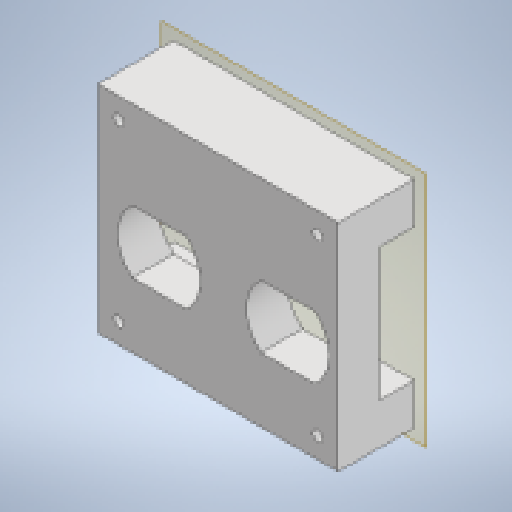
# Autodesk Inventor part: house_V5
Saved by Autodesk Inventor 2023 (Build 270158000, 158)
## iProperties
Created: 2023-03-13
Part Number: house_V5
Material: Generic
Document SubType Name: Modeling
Designer: shrey
Density: 1 g/cm^3
Appearance: Default
Author: shrey
Autodesk Inventor part; units mm, degrees
ref_plane "YZ Plane" through (0, 0, 0) normal (1, 0, 0) x (0, 1, 0)
ref_plane "XZ Plane" through (0, 0, 0) normal (0, 1, 0) x (-1, 0, 0)
ref_plane "XY Plane" through (0, 0, 0) normal (0, 0, 1) x (1, 0, 0)
ref_plane "Work Plane1" through (-29.0856, -229.9846, 23.749) normal (0, 0, 1) x (1, 0, 0)
sketch "Sketch1" plane through (-29.0856, -229.9846, 23.749) normal (0, 0, 1) x (1, 0, 0)
  line L0 (-29.0856, -26.0746) -> (29.0856, -26.0746) construction
  line L1 (29.0856, -26.0746) -> (29.0856, 26.0746) construction
  line L2 (29.0856, 26.0746) -> (-29.0856, 26.0746) construction
  line L3 (-29.0856, 26.0746) -> (-29.0856, -26.0746) construction
  circle A0 centre (24.0856, -21.0746) radius 1.25 construction
  circle A1 centre (-24.0854, -21.0746) radius 1.25 construction
  circle A2 centre (24.0856, 21.0744) radius 1.25 construction
  circle A3 centre (-24.0854, 21.0744) radius 1.25 construction
  arc A4 (23.3986, -10.4091) -> (23.3986, 4.5909) centre (16.7842, -2.9091) ccw construction
  line L4 (10.3986, 4.5909) -> (23.3986, 4.5909) construction
  arc A5 (10.3986, 4.5909) -> (10.3986, -10.4091) centre (17.0129, -2.9091) ccw construction
  line L5 (23.3986, -10.4091) -> (10.3986, -10.4091) construction
  arc A6 (-7.7501, -10.2995) -> (-7.7501, 4.7005) centre (-14.3644, -2.7995) ccw construction
  line L6 (-20.7501, 4.7005) -> (-7.7501, 4.7005) construction
  arc A7 (-20.7501, 4.7005) -> (-20.7501, -10.2995) centre (-14.1357, -2.7995) ccw construction
  line L7 (-7.7501, -10.2995) -> (-20.7501, -10.2995) construction
  spline S0 degree 3 poles (-70.3801, 6.5313) (-70.2603, 6.7214) (-70.0805, 7.0065) (-69.8595, 7.3979) (-69.7007, 7.6952) (-69.5502, 7.9968) (-69.4085, 8.3027) (-69.2764, 8.6129) (-69.155, 8.9274) (-69.046, 9.2463) (-68.95, 9.5696) (-68.8876, 9.8435) (-68.8425, 10.0636) (-68.7948, 10.2255) (-68.7304, 10.3815) (-68.6465, 10.5283) (-68.558, 10.6379) (-68.4781, 10.7171) (-68.4105, 10.7676) (-68.3413, 10.816) (-68.265, 10.8522) (-68.1875, 10.8857) (-68.1054, 10.9055) (-68.0227, 10.9222) (-67.9101, 10.9262) (-67.7698, 10.9236) (-67.6294, 10.9262) (-67.5169, 10.9222) (-67.4341, 10.9055) (-67.352, 10.8857) (-67.2745, 10.8522) (-67.1982, 10.816) (-67.129, 10.7676) (-67.0614, 10.7171) (-66.9815, 10.6379) (-66.8931, 10.5283) (-66.8091, 10.3815) (-66.7447, 10.2255) (-66.6971, 10.0636) (-66.652, 9.8435) (-66.5895, 9.5696) (-66.4936, 9.2463) (-66.3845, 8.9274) (-66.2631, 8.6129) (-66.1311, 8.3027) (-65.9894, 7.9968) (-65.8389, 7.6952) (-65.68, 7.3979) (-65.459, 7.0065) (-65.2792, 6.7214) (-65.1594, 6.5313) knots -1.0784 -1.0784 -1.0784 -1.0784 -1.010995 -0.977291 -0.943586 -0.909882 -0.876178 -0.842474 -0.80877 -0.775067 -0.741365 -0.707665 -0.690816 -0.67397 -0.657123 -0.640284 -0.623449 -0.615023 -0.606598 -0.598176 -0.589749 -0.581327 -0.572901 -0.564477 -0.556053 -0.5392 -0.522347 -0.513923 -0.505499 -0.497074 -0.488651 -0.480225 -0.471802 -0.463377 -0.454951 -0.438116 -0.421277 -0.40443 -0.387584 -0.370735 -0.337035 -0.303333 -0.26963 -0.235926 -0.202222 -0.168518 -0.134814 -0.101109 -0.067405 0 0 0 0 construction
  line L8 (-65.1594, 6.5313) -> (-64.0971, 6.5313) construction
  spline S1 degree 3 poles (-64.0971, 6.5313) (-63.9773, 6.7214) (-63.7975, 7.0065) (-63.5765, 7.3979) (-63.4177, 7.6952) (-63.2672, 7.9968) (-63.1255, 8.3027) (-62.9934, 8.6129) (-62.872, 8.9274) (-62.763, 9.2463) (-62.667, 9.5696) (-62.6046, 9.8435) (-62.5595, 10.0636) (-62.5118, 10.2255) (-62.4474, 10.3815) (-62.3635, 10.5283) (-62.275, 10.6379) (-62.1951, 10.7171) (-62.1275, 10.7676) (-62.0583, 10.816) (-61.982, 10.8522) (-61.9045, 10.8857) (-61.8224, 10.9055) (-61.7397, 10.9222) (-61.6271, 10.9262) (-61.4868, 10.9236) (-61.3464, 10.9262) (-61.2339, 10.9222) (-61.1511, 10.9055) (-61.069, 10.8857) (-60.9915, 10.8522) (-60.9152, 10.816) (-60.846, 10.7676) (-60.7784, 10.7171) (-60.6985, 10.6379) (-60.6101, 10.5283) (-60.5261, 10.3815) (-60.4617, 10.2255) (-60.4141, 10.0636) (-60.369, 9.8435) (-60.3065, 9.5696) (-60.2106, 9.2463) (-60.1015, 8.9274) (-59.9801, 8.6129) (-59.8481, 8.3027) (-59.7064, 7.9968) (-59.5559, 7.6952) (-59.397, 7.3979) (-59.176, 7.0065) (-58.9962, 6.7214) (-58.8764, 6.5313) knots -1.0784 -1.0784 -1.0784 -1.0784 -1.010995 -0.977291 -0.943586 -0.909882 -0.876178 -0.842474 -0.80877 -0.775067 -0.741365 -0.707665 -0.690816 -0.67397 -0.657123 -0.640284 -0.623449 -0.615023 -0.606598 -0.598176 -0.589749 -0.581327 -0.572901 -0.564477 -0.556053 -0.5392 -0.522347 -0.513923 -0.505499 -0.497074 -0.488651 -0.480225 -0.471802 -0.463377 -0.454951 -0.438116 -0.421277 -0.40443 -0.387584 -0.370735 -0.337035 -0.303333 -0.26963 -0.235926 -0.202222 -0.168518 -0.134814 -0.101109 -0.067405 0 0 0 0 construction
  line L9 (-58.8764, 6.5313) -> (-57.8141, 6.5313) construction
  spline S2 degree 3 poles (-57.8141, 6.5313) (-57.6943, 6.7214) (-57.5145, 7.0065) (-57.2935, 7.3979) (-57.1347, 7.6952) (-56.9842, 7.9968) (-56.8425, 8.3027) (-56.7104, 8.6129) (-56.589, 8.9274) (-56.48, 9.2463) (-56.384, 9.5696) (-56.3216, 9.8435) (-56.2765, 10.0636) (-56.2288, 10.2255) (-56.1644, 10.3815) (-56.0805, 10.5283) (-55.992, 10.6379) (-55.9121, 10.7171) (-55.8445, 10.7676) (-55.7753, 10.816) (-55.699, 10.8522) (-55.6215, 10.8857) (-55.5394, 10.9055) (-55.4567, 10.9222) (-55.3441, 10.9262) (-55.2038, 10.9236) (-55.0634, 10.9262) (-54.9509, 10.9222) (-54.8681, 10.9055) (-54.786, 10.8857) (-54.7085, 10.8522) (-54.6322, 10.816) (-54.563, 10.7676) (-54.4954, 10.7171) (-54.4155, 10.6379) (-54.3271, 10.5283) (-54.2431, 10.3815) (-54.1787, 10.2255) (-54.1311, 10.0636) (-54.086, 9.8435) (-54.0235, 9.5696) (-53.9276, 9.2463) (-53.8185, 8.9274) (-53.6971, 8.6129) (-53.5651, 8.3027) (-53.4234, 7.9968) (-53.2729, 7.6952) (-53.114, 7.3979) (-52.893, 7.0065) (-52.7132, 6.7214) (-52.5934, 6.5313) knots -1.0784 -1.0784 -1.0784 -1.0784 -1.010995 -0.977291 -0.943586 -0.909882 -0.876178 -0.842474 -0.80877 -0.775067 -0.741365 -0.707665 -0.690816 -0.67397 -0.657123 -0.640284 -0.623449 -0.615023 -0.606598 -0.598176 -0.589749 -0.581327 -0.572901 -0.564477 -0.556053 -0.5392 -0.522347 -0.513923 -0.505499 -0.497074 -0.488651 -0.480225 -0.471802 -0.463377 -0.454951 -0.438116 -0.421277 -0.40443 -0.387584 -0.370735 -0.337035 -0.303333 -0.26963 -0.235926 -0.202222 -0.168518 -0.134814 -0.101109 -0.067405 0 0 0 0 construction
  line L10 (-52.5934, 6.5313) -> (-51.5311, 6.5313) construction
  spline S3 degree 3 poles (-51.5311, 6.5313) (-51.4113, 6.7214) (-51.2315, 7.0065) (-51.0105, 7.3979) (-50.8517, 7.6952) (-50.7012, 7.9968) (-50.5595, 8.3027) (-50.4274, 8.6129) (-50.306, 8.9274) (-50.197, 9.2463) (-50.101, 9.5696) (-50.0386, 9.8435) (-49.9935, 10.0636) (-49.9458, 10.2255) (-49.8814, 10.3815) (-49.7975, 10.5283) (-49.709, 10.6379) (-49.6291, 10.7171) (-49.5615, 10.7676) (-49.4923, 10.816) (-49.416, 10.8522) (-49.3385, 10.8857) (-49.2564, 10.9055) (-49.1737, 10.9222) (-49.0611, 10.9262) (-48.9208, 10.9236) (-48.7804, 10.9262) (-48.6679, 10.9222) (-48.5851, 10.9055) (-48.503, 10.8857) (-48.4255, 10.8522) (-48.3492, 10.816) (-48.28, 10.7676) (-48.2124, 10.7171) (-48.1325, 10.6379) (-48.0441, 10.5283) (-47.9601, 10.3815) (-47.8957, 10.2255) (-47.8481, 10.0636) (-47.803, 9.8435) (-47.7405, 9.5696) (-47.6446, 9.2463) (-47.5355, 8.9274) (-47.4141, 8.6129) (-47.2821, 8.3027) (-47.1404, 7.9968) (-46.9899, 7.6952) (-46.831, 7.3979) (-46.61, 7.0065) (-46.4302, 6.7214) (-46.3104, 6.5313) knots -1.0784 -1.0784 -1.0784 -1.0784 -1.010995 -0.977291 -0.943586 -0.909882 -0.876178 -0.842474 -0.80877 -0.775067 -0.741365 -0.707665 -0.690816 -0.67397 -0.657123 -0.640284 -0.623449 -0.615023 -0.606598 -0.598176 -0.589749 -0.581327 -0.572901 -0.564477 -0.556053 -0.5392 -0.522347 -0.513923 -0.505499 -0.497074 -0.488651 -0.480225 -0.471802 -0.463377 -0.454951 -0.438116 -0.421277 -0.40443 -0.387584 -0.370735 -0.337035 -0.303333 -0.26963 -0.235926 -0.202222 -0.168518 -0.134814 -0.101109 -0.067405 0 0 0 0 construction
  line L11 (-46.3104, 6.5313) -> (-45.2481, 6.5313) construction
  spline S4 degree 3 poles (-45.2481, 6.5313) (-45.1283, 6.7214) (-44.9485, 7.0065) (-44.7275, 7.3979) (-44.5687, 7.6952) (-44.4182, 7.9968) (-44.2765, 8.3027) (-44.1444, 8.6129) (-44.023, 8.9274) (-43.914, 9.2463) (-43.818, 9.5696) (-43.7556, 9.8435) (-43.7105, 10.0636) (-43.6628, 10.2255) (-43.5984, 10.3815) (-43.5145, 10.5283) (-43.426, 10.6379) (-43.3461, 10.7171) (-43.2785, 10.7676) (-43.2093, 10.816) (-43.133, 10.8522) (-43.0555, 10.8857) (-42.9734, 10.9055) (-42.8907, 10.9222) (-42.7781, 10.9262) (-42.6378, 10.9236) (-42.4974, 10.9262) (-42.3849, 10.9222) (-42.3021, 10.9055) (-42.22, 10.8857) (-42.1425, 10.8522) (-42.0662, 10.816) (-41.997, 10.7676) (-41.9294, 10.7171) (-41.8495, 10.6379) (-41.7611, 10.5283) (-41.6771, 10.3815) (-41.6127, 10.2255) (-41.5651, 10.0636) (-41.52, 9.8435) (-41.4575, 9.5696) (-41.3616, 9.2463) (-41.2525, 8.9274) (-41.1311, 8.6129) (-40.9991, 8.3027) (-40.8574, 7.9968) (-40.7069, 7.6952) (-40.548, 7.3979) (-40.327, 7.0065) (-40.1472, 6.7214) (-40.0274, 6.5313) knots -1.0784 -1.0784 -1.0784 -1.0784 -1.010995 -0.977291 -0.943586 -0.909882 -0.876178 -0.842474 -0.80877 -0.775067 -0.741365 -0.707665 -0.690816 -0.67397 -0.657123 -0.640284 -0.623449 -0.615023 -0.606598 -0.598176 -0.589749 -0.581327 -0.572901 -0.564477 -0.556053 -0.5392 -0.522347 -0.513923 -0.505499 -0.497074 -0.488651 -0.480225 -0.471802 -0.463377 -0.454951 -0.438116 -0.421277 -0.40443 -0.387584 -0.370735 -0.337035 -0.303333 -0.26963 -0.235926 -0.202222 -0.168518 -0.134814 -0.101109 -0.067405 0 0 0 0 construction
  line L12 (-40.0274, 6.5313) -> (-38.9651, 6.5313) construction
  spline S5 degree 3 poles (-38.9651, 6.5313) (-38.8453, 6.7214) (-38.6655, 7.0065) (-38.4445, 7.3979) (-38.2857, 7.6952) (-38.1352, 7.9968) (-37.9935, 8.3027) (-37.8614, 8.6129) (-37.74, 8.9274) (-37.631, 9.2463) (-37.535, 9.5696) (-37.4726, 9.8435) (-37.4275, 10.0636) (-37.3798, 10.2255) (-37.3154, 10.3815) (-37.2315, 10.5283) (-37.143, 10.6379) (-37.0631, 10.7171) (-36.9955, 10.7676) (-36.9263, 10.816) (-36.85, 10.8522) (-36.7725, 10.8857) (-36.6904, 10.9055) (-36.6077, 10.9222) (-36.4951, 10.9262) (-36.3548, 10.9236) (-36.2144, 10.9262) (-36.1019, 10.9222) (-36.0191, 10.9055) (-35.937, 10.8857) (-35.8595, 10.8522) (-35.7832, 10.816) (-35.714, 10.7676) (-35.6464, 10.7171) (-35.5665, 10.6379) (-35.4781, 10.5283) (-35.3941, 10.3815) (-35.3297, 10.2255) (-35.2821, 10.0636) (-35.237, 9.8435) (-35.1745, 9.5696) (-35.0786, 9.2463) (-34.9695, 8.9274) (-34.8481, 8.6129) (-34.7161, 8.3027) (-34.5744, 7.9968) (-34.4239, 7.6952) (-34.265, 7.3979) (-34.044, 7.0065) (-33.8642, 6.7214) (-33.7444, 6.5313) knots -1.0784 -1.0784 -1.0784 -1.0784 -1.010995 -0.977291 -0.943586 -0.909882 -0.876178 -0.842474 -0.80877 -0.775067 -0.741365 -0.707665 -0.690816 -0.67397 -0.657123 -0.640284 -0.623449 -0.615023 -0.606598 -0.598176 -0.589749 -0.581327 -0.572901 -0.564477 -0.556053 -0.5392 -0.522347 -0.513923 -0.505499 -0.497074 -0.488651 -0.480225 -0.471802 -0.463377 -0.454951 -0.438116 -0.421277 -0.40443 -0.387584 -0.370735 -0.337035 -0.303333 -0.26963 -0.235926 -0.202222 -0.168518 -0.134814 -0.101109 -0.067405 0 0 0 0 construction
  line L13 (-33.7444, 6.5313) -> (-32.6821, 6.5313) construction
  spline S6 degree 3 poles (-32.6821, 6.5313) (-32.5623, 6.7214) (-32.3825, 7.0065) (-32.1615, 7.3979) (-32.0027, 7.6952) (-31.8522, 7.9968) (-31.7105, 8.3027) (-31.5784, 8.6129) (-31.457, 8.9274) (-31.348, 9.2463) (-31.252, 9.5696) (-31.1896, 9.8435) (-31.1445, 10.0636) (-31.0968, 10.2255) (-31.0324, 10.3815) (-30.9485, 10.5283) (-30.86, 10.6379) (-30.7801, 10.7171) (-30.7125, 10.7676) (-30.6433, 10.816) (-30.567, 10.8522) (-30.4895, 10.8857) (-30.4074, 10.9055) (-30.3247, 10.9222) (-30.2121, 10.9262) (-30.0718, 10.9236) (-29.9314, 10.9262) (-29.8189, 10.9222) (-29.7361, 10.9055) (-29.654, 10.8857) (-29.5765, 10.8522) (-29.5002, 10.816) (-29.431, 10.7676) (-29.3634, 10.7171) (-29.2835, 10.6379) (-29.1951, 10.5283) (-29.1111, 10.3815) (-29.0467, 10.2255) (-28.9991, 10.0636) (-28.954, 9.8435) (-28.8915, 9.5696) (-28.7956, 9.2463) (-28.6865, 8.9274) (-28.5651, 8.6129) (-28.4331, 8.3027) (-28.2914, 7.9968) (-28.1409, 7.6952) (-27.982, 7.3979) (-27.761, 7.0065) (-27.5812, 6.7214) (-27.4614, 6.5313) knots -1.0784 -1.0784 -1.0784 -1.0784 -1.010995 -0.977291 -0.943586 -0.909882 -0.876178 -0.842474 -0.80877 -0.775067 -0.741365 -0.707665 -0.690816 -0.67397 -0.657123 -0.640284 -0.623449 -0.615023 -0.606598 -0.598176 -0.589749 -0.581327 -0.572901 -0.564477 -0.556053 -0.5392 -0.522347 -0.513923 -0.505499 -0.497074 -0.488651 -0.480225 -0.471802 -0.463377 -0.454951 -0.438116 -0.421277 -0.40443 -0.387584 -0.370735 -0.337035 -0.303333 -0.26963 -0.235926 -0.202222 -0.168518 -0.134814 -0.101109 -0.067405 0 0 0 0 construction
  line L14 (-27.4614, 6.5313) -> (-26.3991, 6.5313) construction
  spline S7 degree 3 poles (-26.3991, 6.5313) (-26.2793, 6.7214) (-26.0995, 7.0065) (-25.8785, 7.3979) (-25.7197, 7.6952) (-25.5692, 7.9968) (-25.4275, 8.3027) (-25.2954, 8.6129) (-25.174, 8.9274) (-25.065, 9.2463) (-24.969, 9.5696) (-24.9066, 9.8435) (-24.8615, 10.0636) (-24.8138, 10.2255) (-24.7494, 10.3815) (-24.6655, 10.5283) (-24.577, 10.6379) (-24.4971, 10.7171) (-24.4295, 10.7676) (-24.3603, 10.816) (-24.284, 10.8522) (-24.2065, 10.8857) (-24.1244, 10.9055) (-24.0417, 10.9222) (-23.9291, 10.9262) (-23.7888, 10.9236) (-23.6484, 10.9262) (-23.5359, 10.9222) (-23.4531, 10.9055) (-23.371, 10.8857) (-23.2935, 10.8522) (-23.2172, 10.816) (-23.148, 10.7676) (-23.0804, 10.7171) (-23.0005, 10.6379) (-22.9121, 10.5283) (-22.8281, 10.3815) (-22.7637, 10.2255) (-22.7161, 10.0636) (-22.671, 9.8435) (-22.6085, 9.5696) (-22.5126, 9.2463) (-22.4035, 8.9274) (-22.2821, 8.6129) (-22.1501, 8.3027) (-22.0084, 7.9968) (-21.8579, 7.6952) (-21.699, 7.3979) (-21.478, 7.0065) (-21.2982, 6.7214) (-21.1784, 6.5313) knots -1.0784 -1.0784 -1.0784 -1.0784 -1.010995 -0.977291 -0.943586 -0.909882 -0.876178 -0.842474 -0.80877 -0.775067 -0.741365 -0.707665 -0.690816 -0.67397 -0.657123 -0.640284 -0.623449 -0.615023 -0.606598 -0.598176 -0.589749 -0.581327 -0.572901 -0.564477 -0.556053 -0.5392 -0.522347 -0.513923 -0.505499 -0.497074 -0.488651 -0.480225 -0.471802 -0.463377 -0.454951 -0.438116 -0.421277 -0.40443 -0.387584 -0.370735 -0.337035 -0.303333 -0.26963 -0.235926 -0.202222 -0.168518 -0.134814 -0.101109 -0.067405 0 0 0 0 construction
  line L15 (-21.1784, 6.5313) -> (-20.1161, 6.5313) construction
  spline S8 degree 3 poles (-20.1161, 6.5313) (-19.9963, 6.7214) (-19.8165, 7.0065) (-19.5955, 7.3979) (-19.4367, 7.6952) (-19.2862, 7.9968) (-19.1445, 8.3027) (-19.0124, 8.6129) (-18.891, 8.9274) (-18.782, 9.2463) (-18.686, 9.5696) (-18.6236, 9.8435) (-18.5785, 10.0636) (-18.5308, 10.2255) (-18.4664, 10.3815) (-18.3825, 10.5283) (-18.294, 10.6379) (-18.2141, 10.7171) (-18.1465, 10.7676) (-18.0773, 10.816) (-18.001, 10.8522) (-17.9235, 10.8857) (-17.8414, 10.9055) (-17.7587, 10.9222) (-17.6461, 10.9262) (-17.5058, 10.9236) (-17.3654, 10.9262) (-17.2529, 10.9222) (-17.1701, 10.9055) (-17.088, 10.8857) (-17.0105, 10.8522) (-16.9342, 10.816) (-16.865, 10.7676) (-16.7974, 10.7171) (-16.7175, 10.6379) (-16.6291, 10.5283) (-16.5451, 10.3815) (-16.4807, 10.2255) (-16.4331, 10.0636) (-16.388, 9.8435) (-16.3255, 9.5696) (-16.2296, 9.2463) (-16.1205, 8.9274) (-15.9991, 8.6129) (-15.8671, 8.3027) (-15.7254, 7.9968) (-15.5749, 7.6952) (-15.416, 7.3979) (-15.195, 7.0065) (-15.0152, 6.7214) (-14.8954, 6.5313) knots -1.0784 -1.0784 -1.0784 -1.0784 -1.010995 -0.977291 -0.943586 -0.909882 -0.876178 -0.842474 -0.80877 -0.775067 -0.741365 -0.707665 -0.690816 -0.67397 -0.657123 -0.640284 -0.623449 -0.615023 -0.606598 -0.598176 -0.589749 -0.581327 -0.572901 -0.564477 -0.556053 -0.5392 -0.522347 -0.513923 -0.505499 -0.497074 -0.488651 -0.480225 -0.471802 -0.463377 -0.454951 -0.438116 -0.421277 -0.40443 -0.387584 -0.370735 -0.337035 -0.303333 -0.26963 -0.235926 -0.202222 -0.168518 -0.134814 -0.101109 -0.067405 0 0 0 0 construction
  line L16 (-14.8954, 6.5313) -> (-13.8331, 6.5313) construction
  spline S9 degree 3 poles (-13.8331, 6.5313) (-13.7133, 6.7214) (-13.5335, 7.0065) (-13.3125, 7.3979) (-13.1537, 7.6952) (-13.0032, 7.9968) (-12.8615, 8.3027) (-12.7294, 8.6129) (-12.608, 8.9274) (-12.499, 9.2463) (-12.403, 9.5696) (-12.3406, 9.8435) (-12.2955, 10.0636) (-12.2478, 10.2255) (-12.1834, 10.3815) (-12.0995, 10.5283) (-12.011, 10.6379) (-11.9311, 10.7171) (-11.8635, 10.7676) (-11.7943, 10.816) (-11.718, 10.8522) (-11.6405, 10.8857) (-11.5584, 10.9055) (-11.4757, 10.9222) (-11.3631, 10.9262) (-11.2228, 10.9236) (-11.0824, 10.9262) (-10.9699, 10.9222) (-10.8871, 10.9055) (-10.805, 10.8857) (-10.7275, 10.8522) (-10.6512, 10.816) (-10.582, 10.7676) (-10.5144, 10.7171) (-10.4345, 10.6379) (-10.3461, 10.5283) (-10.2621, 10.3815) (-10.1977, 10.2255) (-10.1501, 10.0636) (-10.105, 9.8435) (-10.0425, 9.5696) (-9.9466, 9.2463) (-9.8375, 8.9274) (-9.7161, 8.6129) (-9.5841, 8.3027) (-9.4424, 7.9968) (-9.2919, 7.6952) (-9.133, 7.3979) (-8.912, 7.0065) (-8.7322, 6.7214) (-8.6124, 6.5313) knots -1.0784 -1.0784 -1.0784 -1.0784 -1.010995 -0.977291 -0.943586 -0.909882 -0.876178 -0.842474 -0.80877 -0.775067 -0.741365 -0.707665 -0.690816 -0.67397 -0.657123 -0.640284 -0.623449 -0.615023 -0.606598 -0.598176 -0.589749 -0.581327 -0.572901 -0.564477 -0.556053 -0.5392 -0.522347 -0.513923 -0.505499 -0.497074 -0.488651 -0.480225 -0.471802 -0.463377 -0.454951 -0.438116 -0.421277 -0.40443 -0.387584 -0.370735 -0.337035 -0.303333 -0.26963 -0.235926 -0.202222 -0.168518 -0.134814 -0.101109 -0.067405 0 0 0 0 construction
  line L17 (-8.6124, 6.5313) -> (-7.5501, 6.5313) construction
  spline S10 degree 3 poles (-7.5501, 6.5313) (-7.4303, 6.7214) (-7.2505, 7.0065) (-7.0295, 7.3979) (-6.8707, 7.6952) (-6.7202, 7.9968) (-6.5785, 8.3027) (-6.4464, 8.6129) (-6.325, 8.9274) (-6.216, 9.2463) (-6.12, 9.5696) (-6.0576, 9.8435) (-6.0125, 10.0636) (-5.9648, 10.2255) (-5.9004, 10.3815) (-5.8165, 10.5283) (-5.728, 10.6379) (-5.6481, 10.7171) (-5.5805, 10.7676) (-5.5113, 10.816) (-5.435, 10.8522) (-5.3575, 10.8857) (-5.2754, 10.9055) (-5.1927, 10.9222) (-5.0801, 10.9262) (-4.9398, 10.9236) (-4.7994, 10.9262) (-4.6869, 10.9222) (-4.6041, 10.9055) (-4.522, 10.8857) (-4.4445, 10.8522) (-4.3682, 10.816) (-4.299, 10.7676) (-4.2314, 10.7171) (-4.1515, 10.6379) (-4.0631, 10.5283) (-3.9791, 10.3815) (-3.9147, 10.2255) (-3.8671, 10.0636) (-3.822, 9.8435) (-3.7595, 9.5696) (-3.6636, 9.2463) (-3.5545, 8.9274) (-3.4331, 8.6129) (-3.3011, 8.3027) (-3.1594, 7.9968) (-3.0089, 7.6952) (-2.85, 7.3979) (-2.629, 7.0065) (-2.4492, 6.7214) (-2.3294, 6.5313) knots -1.0784 -1.0784 -1.0784 -1.0784 -1.010995 -0.977291 -0.943586 -0.909882 -0.876178 -0.842474 -0.80877 -0.775067 -0.741365 -0.707665 -0.690816 -0.67397 -0.657123 -0.640284 -0.623449 -0.615023 -0.606598 -0.598176 -0.589749 -0.581327 -0.572901 -0.564477 -0.556053 -0.5392 -0.522347 -0.513923 -0.505499 -0.497074 -0.488651 -0.480225 -0.471802 -0.463377 -0.454951 -0.438116 -0.421277 -0.40443 -0.387584 -0.370735 -0.337035 -0.303333 -0.26963 -0.235926 -0.202222 -0.168518 -0.134814 -0.101109 -0.067405 0 0 0 0 construction
  line L18 (-2.3294, 6.5313) -> (-1.2671, 6.5313) construction
  spline S11 degree 3 poles (-1.2671, 6.5313) (-1.1473, 6.7214) (-0.9675, 7.0065) (-0.7465, 7.3979) (-0.5877, 7.6952) (-0.4372, 7.9968) (-0.2955, 8.3027) (-0.1634, 8.6129) (-0.042, 8.9274) (0.067, 9.2463) (0.163, 9.5696) (0.2254, 9.8435) (0.2705, 10.0636) (0.3182, 10.2255) (0.3826, 10.3815) (0.4665, 10.5283) (0.555, 10.6379) (0.6349, 10.7171) (0.7025, 10.7676) (0.7717, 10.816) (0.848, 10.8522) (0.9255, 10.8857) (1.0076, 10.9055) (1.0903, 10.9222) (1.2029, 10.9262) (1.3432, 10.9236) (1.4836, 10.9262) (1.5961, 10.9222) (1.6789, 10.9055) (1.761, 10.8857) (1.8385, 10.8522) (1.9148, 10.816) (1.984, 10.7676) (2.0516, 10.7171) (2.1315, 10.6379) (2.2199, 10.5283) (2.3039, 10.3815) (2.3683, 10.2255) (2.4159, 10.0636) (2.461, 9.8435) (2.5235, 9.5696) (2.6194, 9.2463) (2.7285, 8.9274) (2.8499, 8.6129) (2.9819, 8.3027) (3.1236, 7.9968) (3.2741, 7.6952) (3.433, 7.3979) (3.654, 7.0065) (3.8338, 6.7214) (3.9536, 6.5313) knots -1.0784 -1.0784 -1.0784 -1.0784 -1.010995 -0.977291 -0.943586 -0.909882 -0.876178 -0.842474 -0.80877 -0.775067 -0.741365 -0.707665 -0.690816 -0.67397 -0.657123 -0.640284 -0.623449 -0.615023 -0.606598 -0.598176 -0.589749 -0.581327 -0.572901 -0.564477 -0.556053 -0.5392 -0.522347 -0.513923 -0.505499 -0.497074 -0.488651 -0.480225 -0.471802 -0.463377 -0.454951 -0.438116 -0.421277 -0.40443 -0.387584 -0.370735 -0.337035 -0.303333 -0.26963 -0.235926 -0.202222 -0.168518 -0.134814 -0.101109 -0.067405 0 0 0 0 construction
  line L19 (3.9536, 6.5313) -> (5.0159, 6.5313) construction
  spline S12 degree 3 poles (5.0159, 6.5313) (5.1357, 6.7214) (5.3155, 7.0065) (5.5365, 7.3979) (5.6953, 7.6952) (5.8458, 7.9968) (5.9875, 8.3027) (6.1196, 8.6129) (6.241, 8.9274) (6.35, 9.2463) (6.446, 9.5696) (6.5084, 9.8435) (6.5535, 10.0636) (6.6012, 10.2255) (6.6656, 10.3815) (6.7495, 10.5283) (6.838, 10.6379) (6.9179, 10.7171) (6.9855, 10.7676) (7.0547, 10.816) (7.131, 10.8522) (7.2085, 10.8857) (7.2906, 10.9055) (7.3733, 10.9222) (7.4859, 10.9262) (7.6262, 10.9236) (7.7666, 10.9262) (7.8791, 10.9222) (7.9619, 10.9055) (8.044, 10.8857) (8.1215, 10.8522) (8.1978, 10.816) (8.267, 10.7676) (8.3346, 10.7171) (8.4145, 10.6379) (8.5029, 10.5283) (8.5869, 10.3815) (8.6513, 10.2255) (8.6989, 10.0636) (8.744, 9.8435) (8.8065, 9.5696) (8.9024, 9.2463) (9.0115, 8.9274) (9.1329, 8.6129) (9.2649, 8.3027) (9.4066, 7.9968) (9.5571, 7.6952) (9.716, 7.3979) (9.937, 7.0065) (10.1168, 6.7214) (10.2366, 6.5313) knots -1.0784 -1.0784 -1.0784 -1.0784 -1.010995 -0.977291 -0.943586 -0.909882 -0.876178 -0.842474 -0.80877 -0.775067 -0.741365 -0.707665 -0.690816 -0.67397 -0.657123 -0.640284 -0.623449 -0.615023 -0.606598 -0.598176 -0.589749 -0.581327 -0.572901 -0.564477 -0.556053 -0.5392 -0.522347 -0.513923 -0.505499 -0.497074 -0.488651 -0.480225 -0.471802 -0.463377 -0.454951 -0.438116 -0.421277 -0.40443 -0.387584 -0.370735 -0.337035 -0.303333 -0.26963 -0.235926 -0.202222 -0.168518 -0.134814 -0.101109 -0.067405 0 0 0 0 construction
  line L20 (10.2366, 6.5313) -> (11.2989, 6.5313) construction
  spline S13 degree 3 poles (11.2989, 6.5313) (11.4187, 6.7214) (11.5985, 7.0065) (11.8195, 7.3979) (11.9783, 7.6952) (12.1288, 7.9968) (12.2705, 8.3027) (12.4026, 8.6129) (12.524, 8.9274) (12.633, 9.2463) (12.729, 9.5696) (12.7914, 9.8435) (12.8365, 10.0636) (12.8842, 10.2255) (12.9486, 10.3815) (13.0325, 10.5283) (13.121, 10.6379) (13.2009, 10.7171) (13.2685, 10.7676) (13.3377, 10.816) (13.414, 10.8522) (13.4915, 10.8857) (13.5736, 10.9055) (13.6563, 10.9222) (13.7689, 10.9262) (13.9092, 10.9236) (14.0496, 10.9262) (14.1621, 10.9222) (14.2449, 10.9055) (14.327, 10.8857) (14.4045, 10.8522) (14.4808, 10.816) (14.55, 10.7676) (14.6176, 10.7171) (14.6975, 10.6379) (14.7859, 10.5283) (14.8699, 10.3815) (14.9343, 10.2255) (14.9819, 10.0636) (15.027, 9.8435) (15.0895, 9.5696) (15.1854, 9.2463) (15.2945, 8.9274) (15.4159, 8.6129) (15.5479, 8.3027) (15.6896, 7.9968) (15.8401, 7.6952) (15.999, 7.3979) (16.22, 7.0065) (16.3998, 6.7214) (16.5196, 6.5313) knots -1.0784 -1.0784 -1.0784 -1.0784 -1.010995 -0.977291 -0.943586 -0.909882 -0.876178 -0.842474 -0.80877 -0.775067 -0.741365 -0.707665 -0.690816 -0.67397 -0.657123 -0.640284 -0.623449 -0.615023 -0.606598 -0.598176 -0.589749 -0.581327 -0.572901 -0.564477 -0.556053 -0.5392 -0.522347 -0.513923 -0.505499 -0.497074 -0.488651 -0.480225 -0.471802 -0.463377 -0.454951 -0.438116 -0.421277 -0.40443 -0.387584 -0.370735 -0.337035 -0.303333 -0.26963 -0.235926 -0.202222 -0.168518 -0.134814 -0.101109 -0.067405 0 0 0 0 construction
  line L21 (16.5196, 6.5313) -> (17.5819, 6.5313) construction
  spline S14 degree 3 poles (17.5819, 6.5313) (17.7017, 6.7214) (17.8815, 7.0065) (18.1025, 7.3979) (18.2613, 7.6952) (18.4118, 7.9968) (18.5535, 8.3027) (18.6856, 8.6129) (18.807, 8.9274) (18.916, 9.2463) (19.012, 9.5696) (19.0744, 9.8435) (19.1195, 10.0636) (19.1672, 10.2255) (19.2316, 10.3815) (19.3155, 10.5283) (19.404, 10.6379) (19.4839, 10.7171) (19.5515, 10.7676) (19.6207, 10.816) (19.697, 10.8522) (19.7745, 10.8857) (19.8566, 10.9055) (19.9393, 10.9222) (20.0519, 10.9262) (20.1922, 10.9236) (20.3326, 10.9262) (20.4451, 10.9222) (20.5279, 10.9055) (20.61, 10.8857) (20.6875, 10.8522) (20.7638, 10.816) (20.833, 10.7676) (20.9006, 10.7171) (20.9805, 10.6379) (21.0689, 10.5283) (21.1529, 10.3815) (21.2173, 10.2255) (21.2649, 10.0636) (21.31, 9.8435) (21.3725, 9.5696) (21.4684, 9.2463) (21.5775, 8.9274) (21.6989, 8.6129) (21.8309, 8.3027) (21.9726, 7.9968) (22.1231, 7.6952) (22.282, 7.3979) (22.503, 7.0065) (22.6828, 6.7214) (22.8026, 6.5313) knots -1.0784 -1.0784 -1.0784 -1.0784 -1.010995 -0.977291 -0.943586 -0.909882 -0.876178 -0.842474 -0.80877 -0.775067 -0.741365 -0.707665 -0.690816 -0.67397 -0.657123 -0.640284 -0.623449 -0.615023 -0.606598 -0.598176 -0.589749 -0.581327 -0.572901 -0.564477 -0.556053 -0.5392 -0.522347 -0.513923 -0.505499 -0.497074 -0.488651 -0.480225 -0.471802 -0.463377 -0.454951 -0.438116 -0.421277 -0.40443 -0.387584 -0.370735 -0.337035 -0.303333 -0.26963 -0.235926 -0.202222 -0.168518 -0.134814 -0.101109 -0.067405 0 0 0 0 construction
  line L22 (22.8026, 6.5313) -> (23.8649, 6.5313) construction
  spline S15 degree 3 poles (23.8649, 6.5313) (24.118, 6.9328) (24.695, 7.848) (25.4194, 9.839) (25.372, 10.1863) (25.6994, 10.6689) (25.8061, 10.7491) (25.9097, 10.8187) (26.0062, 10.8786) (26.2998, 10.9373) (26.4357, 10.9246) (26.6859, 10.9255) (26.7966, 10.923) (27.0207, 10.8327) (27.1144, 10.7723) (27.2536, 10.6564) (27.315, 10.574) (27.4239, 10.4156) (27.4798, 10.2877) (27.5764, 9.9711) (27.5919, 9.8101) (28.0686, 8.0931) (28.9099, 6.81) (29.0856, 6.5313) knots 0 0 0 0 0.142394 0.142394 0.262557 0.262557 0.314666 0.314666 0.34653 0.34653 0.372217 0.372217 0.394622 0.394622 0.411062 0.411062 0.432958 0.432958 0.48678 0.48678 0.562983 0.562983 0.900876 0.900876 0.900876 0.900876 construction
  line L23 (29.0856, 6.5313) -> (29.0856, 15.9246) construction
  line L24 (29.0856, 15.9246) -> (-70.9144, 15.9246) construction
  line L25 (-70.9144, 15.9246) -> (-70.9144, 6.5313) construction
  line L26 (-70.9144, 6.5313) -> (-70.3801, 6.5313) construction
  arc A8 (10.3609, 4.6909) -> (10.3609, -10.5091) centre (17.0129, -2.9091) ccw
  line L27 (10.3609, 4.6909) -> (23.4363, 4.6909)
  arc A9 (23.4363, -10.5091) -> (23.4363, 4.6909) centre (16.7842, -2.9091) ccw
  line L28 (23.4363, -10.5091) -> (10.3609, -10.5091)
  arc A10 (-7.7124, -10.3995) -> (-7.7124, 4.8005) centre (-14.3644, -2.7995) ccw
  line L29 (-7.7124, -10.3995) -> (-20.7878, -10.3995)
  arc A11 (-20.7878, 4.8005) -> (-20.7878, -10.3995) centre (-14.1357, -2.7995) ccw
  line L30 (-20.7878, 4.8005) -> (-7.7124, 4.8005)
  line L31 (29.0856, 26.0746) -> (19.0856, 26.0746)
  line L32 (19.0856, 26.0746) -> (19.0856, 16.0746)
  line L33 (19.0856, 16.0746) -> (29.0856, 16.0746)
  line L34 (29.0856, 16.0746) -> (29.0856, 26.0746)
  circle A12 centre (24.0856, 21.0744) radius 1.25
  line L35 (19.0856, -26.0744) -> (29.0856, -26.0744)
  line L36 (29.0856, -26.0744) -> (29.0856, -16.0744)
  line L37 (19.0856, -16.0744) -> (19.0856, -26.0744)
  line L38 (29.0856, -16.0744) -> (19.0856, -16.0744)
  circle A13 centre (24.0856, -21.0746) radius 1.25
  line L39 (-29.0854, 16.0746) -> (-19.0854, 16.0746)
  line L40 (-19.0854, 16.0746) -> (-19.0854, 26.0746)
  line L41 (-29.0854, 26.0746) -> (-29.0854, 16.0746)
  line L42 (-19.0854, 26.0746) -> (-29.0854, 26.0746)
  circle A14 centre (-24.0854, 21.0744) radius 1.25
  line L43 (-29.0854, -26.0744) -> (-19.0854, -26.0744)
  line L44 (-19.0854, -26.0744) -> (-19.0854, -16.0744)
  line L45 (-29.0854, -16.0744) -> (-29.0854, -26.0744)
  line L46 (-19.0854, -16.0744) -> (-29.0854, -16.0744)
  circle A15 centre (-24.0854, -21.0746) radius 1.25
  line L47 (19.0856, 16.0746) -> (-19.0854, 16.0746)
  line L48 (-19.0854, 16.0746) -> (-19.0854, 26.0746)
  line L49 (-19.0854, 26.0746) -> (19.0856, 26.0746)
  line L50 (19.0856, 26.0746) -> (19.0856, 16.0746)
  point P0 (29.0856, 229.9846)
  point P1 (-19.0854, 16.0746)
  dimension "d0" = 0.1
  dimension "d1" = 0.1
  dimension "d2" = 10
  dimension "d3" = 10
  dimension "d6" = 42.149
  dimension "d9" = 48.171
  constraints: 48 end point, 8 centre point, 8 point on circle, 4 parallel, 3 horizontal, 2 perpendicular, 1 coincident, 1 concentric, 1 vertical, 36 other
  measures "d0" radial gap between concentric circles of A5 A8
  measures "d1" radial gap between concentric circles of A6 A10
  measures "d2" distance of L33.end L32.end
  measures "d3" distance of L32.end L31.end
  measures "d6" distance of L32.end L35.start
  measures "d9" distance of L32.end L39.start
extrude "Extrusion1" add sketch "Sketch1" along normal blind 8.3 contours L34 L33 L32 L31 | L32 L47 L40 L49 | L40 L39 L41 L42 | L37 L38 L36 L35 | L45 L46 L44 L43
sketch "Sketch2" plane through (-29.0856, -229.9846, 32.049) normal (0, 0, 1) x (1, 0, 0)
  line L0 (23.4363, -10.5091) -> (10.3609, -10.5091) projected
  arc A0 (10.3609, 4.6909) -> (10.3609, -10.5091) centre (17.0129, -2.9091) ccw projected
  line L1 (10.3609, 4.6909) -> (23.4363, 4.6909) projected
  arc A1 (23.4363, -10.5091) -> (23.4363, 4.6909) centre (16.7842, -2.9091) ccw projected
  arc A2 (-7.7124, -10.3995) -> (-7.7124, 4.8005) centre (-14.3644, -2.7995) ccw projected
  line L2 (-20.7878, 4.8005) -> (-7.7124, 4.8005) projected
  arc A3 (-20.7878, 4.8005) -> (-20.7878, -10.3995) centre (-14.1357, -2.7995) ccw projected
  line L3 (-7.7124, -10.3995) -> (-20.7878, -10.3995) projected
  line L4 (29.0856, -26.0744) -> (29.0856, -16.0744) projected
  line L5 (-29.0854, 26.0746) -> (-29.0854, 16.0746) projected
  line L6 (29.0856, -26.0744) -> (-29.0854, -26.0744)
  line L7 (-29.0854, -26.0744) -> (-29.0854, 26.0746)
  line L8 (-29.0854, 26.0746) -> (29.0856, 26.0746)
  line L9 (29.0856, 26.0746) -> (29.0856, -26.0744)
  circle A4 centre (24.0856, -21.0746) radius 1.25 projected
  circle A5 centre (-24.0854, -21.0746) radius 1.25 projected
  circle A6 centre (-24.0854, 21.0744) radius 1.25 projected
  circle A7 centre (24.0856, 21.0744) radius 1.25 projected
  point P0 (29.0856, 229.9846)
  constraints: 8 end point, 2 parallel, 1 horizontal, 1 perpendicular
extrude "Extrusion2" add sketch "Sketch2" along normal blind 10
ref_plane "Work Plane2" through (-29.0856, -229.9846, 38.549) normal (0, 0, 1) x (1, 0, 0)
sketch "Sketch3" plane through (-29.0856, -229.9846, 38.549) normal (0, 0, 1) x (1, 0, 0)
  circle A0 centre (24.0856, -21.0746) radius 2.915 projected
  circle A1 centre (24.0856, -21.0746) radius 3.415
  line L0 (29.0856, -26.0744) -> (29.0856, 26.0746) construction
  line L1 (29.0856, 26.0746) -> (-29.0854, 26.0746) construction
  line L2 (-29.0854, 26.0746) -> (-29.0854, -26.0744) construction
  line L3 (-29.0854, -26.0744) -> (29.0856, -26.0744) construction
  circle A2 centre (24.0856, -21.0746) radius 1.25 construction
  circle A3 centre (-24.0854, -21.0746) radius 1.25 construction
  circle A4 centre (-24.0854, 21.0744) radius 1.25 construction
  circle A5 centre (24.0856, 21.0744) radius 1.25 construction
  line L4 (-20.7878, 4.8005) -> (-7.7124, 4.8005) construction
  arc A6 (-7.7124, -10.3995) -> (-7.7124, 4.8005) centre (-14.3644, -2.7995) ccw construction
  line L5 (-7.7124, -10.3995) -> (-20.7878, -10.3995) construction
  arc A7 (-20.7878, 4.8005) -> (-20.7878, -10.3995) centre (-14.1357, -2.7995) ccw construction
  line L6 (10.3609, 4.6909) -> (23.4363, 4.6909) construction
  arc A8 (23.4363, -10.5091) -> (23.4363, 4.6909) centre (16.7842, -2.9091) ccw construction
  line L7 (23.4363, -10.5091) -> (10.3609, -10.5091) construction
  arc A9 (10.3609, 4.6909) -> (10.3609, -10.5091) centre (17.0129, -2.9091) ccw construction
  circle A10 centre (24.0856, 21.0744) radius 3.415
  circle A11 centre (-24.0854, -21.0746) radius 3.415
  circle A12 centre (-24.0854, 21.0744) radius 3.415
  point P0 (29.0856, 229.9846)
  dimension "d17" = 0.5
  dimension "d20" = 42.149
  dimension "d23" = 48.171
  constraints: 4 centre point, 1 horizontal, 1 vertical, 6 other
  measures "d17" radial gap between concentric circles of A0 A1
  measures "d20" distance of A0.centre A10.centre
  measures "d23" distance of A0.centre A11.centre
extrude "Extrusion3" cut sketch "Sketch3" along normal blind 30.75 contours A0 | A1 | A10 | A11 | A12
body "Solid1"
